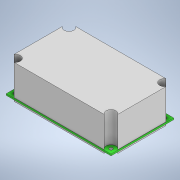
# Autodesk Inventor part: netzteil_12V
Saved by Autodesk Inventor 2021 (Build 250183000, 183)
## iProperties
Created: 2021-07-14
Part Number: netzteil_12V
Material: Generisch
Document SubType Name: Modeling
Designer: Simon
Density: 1 g/cm^3
Appearance: Vorgabe
Author: Simon
Autodesk Inventor part; units mm, degrees
ref_plane "YZ Plane" through (0, 0, 0) normal (1, 0, 0) x (0, 1, 0)
ref_plane "XZ Plane" through (0, 0, 0) normal (0, 1, 0) x (-1, 0, 0)
ref_plane "XY Plane" through (0, 0, 0) normal (0, 0, 1) x (1, 0, 0)
sketch "Skizze1" plane through (0, 0, 0) normal (0, 1, 0) x (-1, 0, 0)
  line L0 (63.5, -38) -> (-63.5, -38)
  line L1 (-63.5, -38) -> (-63.5, 38)
  line L2 (-63.5, 38) -> (63.5, 38)
  line L3 (63.5, 38) -> (63.5, -38)
  point P0 (0, 0)
  point P1 (0, -38)
  point P2 (63.5, 0)
  dimension "d0" = 76
  dimension "d1" = 127
  constraints: 8 end point, 2 midpoint, 2 parallel, 1 horizontal, 1 horizontal alignment, 1 perpendicular, 1 vertical alignment
  measures "d0" distance between parallel lines of L2 L0
  measures "d1" distance between parallel lines of L3 L1
extrude "Extrusion1" add sketch "Skizze1" along normal blind 2
sketch "Skizze2" plane through (0, 2, 0) normal (0, 1, 0) x (1, 0, 0)
  circle A0 centre (-58, 32.5) radius 2
  circle A1 centre (-58, -32.5) radius 2
  circle A2 centre (58, -32.5) radius 2
  circle A3 centre (58, 32.5) radius 2
  point P0 (0, 0)
  dimension "d4" = 4
  dimension "d5" = 4
  dimension "d6" = 4
  dimension "d7" = 4
  dimension "d8" = 116
  dimension "d9" = 58
  dimension "d10" = 65
  dimension "d11" = 32.5
  constraints: 4 centre point, 2 horizontal alignment, 2 vertical alignment
  measures "d4" diameter of A0
  measures "d5" diameter of A1
  measures "d6" diameter of A2
  measures "d7" diameter of A3
  measures "d8" distance of A3.centre A0.centre
  measures "d9" horizontal distance of point (0, 0) A0.centre
  measures "d10" distance of A1.centre A0.centre
  measures "d11" vertical distance of A0.centre point (0, 0)
extrude "Extrusion2" cut sketch "Skizze2" against normal through all
sketch "Skizze4" plane through (0, 2, 0) normal (0, 1, 0) x (1, 0, 0)
  line L0 (-54.6834, 37.5) -> (54.6834, 37.5)
  line L1 (63, 29.1834) -> (63, -29.1834)
  line L2 (54.6834, -37.5) -> (-54.6834, -37.5)
  line L3 (-63, -29.1834) -> (-63, 29.1834)
  line L4 (63.5, -38) -> (63.5, 38) projected
  line L5 (63.5, 38) -> (-63.5, 38) projected
  line L6 (-63.5, -38) -> (63.5, -38) projected
  line L7 (-63.5, 38) -> (-63.5, -38) projected
  circle A0 centre (-58, 32.5) radius 2 projected
  circle A1 centre (-58, -32.5) radius 2 projected
  arc A2 (-54.6834, -37.5) -> (-63, -29.1834) centre (-58, -32.5) ccw
  circle A3 centre (58, -32.5) radius 2 projected
  arc A4 (63, -29.1834) -> (54.6834, -37.5) centre (58, -32.5) ccw
  arc A5 (54.6834, 37.5) -> (63, 29.1834) centre (58, 32.5) ccw
  circle A6 centre (58, 32.5) radius 2 projected
  arc A7 (-63, 29.1834) -> (-54.6834, 37.5) centre (-58, 32.5) ccw
  point P0 (0, 0)
  point P1 (60.3979, -38)
  point P2 (63.5, -34.8979)
  point P3 (-60.3979, -38)
  dimension "d14" = 0.5
  dimension "d15" = 0.5
  dimension "d16" = 0.5
  dimension "d17" = 0.5
  dimension "d19" = 6
  dimension "d21" = 6
  dimension "d22" = 6
  dimension "d27" = 6
  constraints: 9 point on circle, 8 end point, 4 centre point, 4 coincident, 3 point on line, 2 parallel, 1 horizontal, 1 perpendicular
  measures "d14" distance between parallel lines of L4 L1
  measures "d15" distance between parallel lines of L5 L0
  measures "d16" distance between parallel lines of L6 L2
  measures "d17" distance between parallel lines of L7 L3
  measures "d19" radius of A5
  measures "d21" radius of A4
  measures "d22" radius of A2
  measures "d27" radius of A7
extrude "Extrusion3" add sketch "Skizze4" along normal blind 37 and the other way blind 4 contours L0 A5 L1 A4 L2 A2 L3 A7
equation "\"d5\" = d4"
equation "\"d6\" = d4"
equation "\"d7\" = d4"
equation "\"d9\" = 0.5 * d8"
equation "\"d11\" = 0.5 * d10"
equation "\"d14\" = d15"
equation "\"d16\" = d15"
equation "\"d17\" = d15"
equation "\"d19\" = d20"
equation "\"d21\" = d20"
equation "\"d22\" = d27"
equation "\"d20\" = 6"
